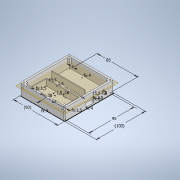
# Autodesk Inventor part: Senzor-case-new
Saved by Autodesk Inventor 2022 (Build 260153000, 153)
## iProperties
Created: 2023-05-16
Part Number: Senzor-case-new
Material: Všeobecné
Document SubType Name: Modeling
Designer: Tada
Density: 1 g/cm^3
Appearance: Výchozí
Author: Tada
Autodesk Inventor part; units mm, degrees
ref_plane "YZ Plane" through (0, 0, 0) normal (1, 0, 0) x (0, 1, 0)
ref_plane "XZ Plane" through (0, 0, 0) normal (0, 1, 0) x (-1, 0, 0)
ref_plane "XY Plane" through (0, 0, 0) normal (0, 0, 1) x (1, 0, 0)
sketch "Náčrt1" plane through (0, 0, 0) normal (0, 1, 0) x (-1, 0, 0)
  line L0 (0, 0) -> (-85, 0)
  line L1 (-85, 0) -> (-85, -95)
  line L2 (-85, -95) -> (0, -95)
  line L3 (0, -95) -> (0, 0)
  line L4 (4, 4) -> (-89, 4)
  line L5 (-89, 4) -> (-89, -99)
  line L6 (-89, -99) -> (4, -99)
  line L7 (4, -99) -> (4, 4)
  line L8 (0, 0) -> (-68, 0)
  line L9 (0, -38) -> (0, 0)
  line L10 (0, 0) -> (-69.5, 0)
  line L11 (0, -39.5) -> (0, 0)
  line L12 (0, -57.5) -> (-69.5, -57.5)
  line L13 (-85, -57.5) -> (-85, -59)
  line L14 (-69.5, -59) -> (0, -59)
  line L15 (0, -59) -> (0, -57.5)
  line L16 (-69.5, -57.5) -> (-69.5, -59)
  circle A0 centre (-77, -71.5) radius 1.25
  circle A1 centre (-77, -87) radius 1.25
  line L17 (0, 0) -> (-68, 0)
  line L18 (0, -38) -> (0, 0)
  line L19 (-7, 0) -> (-78, 0)
  line L20 (-78, 0) -> (-78, -39.5)
  line L21 (-78, -39.5) -> (-7, -39.5)
  line L22 (-7, -39.5) -> (-7, 0)
  line L23 (-8.5, 0) -> (-76.5, 0)
  line L24 (-76.5, 0) -> (-76.5, -38)
  line L25 (-76.5, -38) -> (-8.5, -38)
  line L26 (-8.5, -38) -> (-8.5, 0)
  point P0 (0, -59)
  dimension "d0" = 4
  dimension "d1" = 4
  dimension "d2" = 4
  dimension "d3" = 4
  dimension "d4" = 85
  dimension "d5" = 95
  dimension "d10" = 1.5
  dimension "d12" = 69.5
  dimension "d13" = 2.5
  dimension "d14" = 2.5
  dimension "d15" = 15.5
  dimension "d16" = 8
  dimension "d17" = 8
  dimension "d18" = 8
  dimension "d89" = 1.5
  dimension "d90" = 1.5
  dimension "d91" = 18
  dimension "d92" = 68
  dimension "d93" = 38
  dimension "d94" = 1.5
  dimension "d95" = 7
  dimension "d105" = 93
  dimension "d106" = 103
  constraints: 54 end point, 9 parallel, 7 horizontal, 6 point on line, 5 perpendicular, 2 centre point, 1 vertical
  measures "d0" distance between parallel lines of L7 L3
  measures "d1" distance between parallel lines of L6 L2
  measures "d2" distance between parallel lines of L1 L5
  measures "d3" distance between parallel lines of L4 L0
  measures "d4" distance of L1.end L2.end
  measures "d5" distance of L0.end L1.end
  measures "d10" distance between parallel lines of L12 L14
  measures "d12" distance between parallel lines of L3 L16
  measures "d13" diameter of A1
  measures "d14" diameter of A0
  measures "d15" distance of A1.centre A0.centre
  measures "d16" distance from line of L1 A1.centre
  measures "d17" distance from line of L2 A1.centre
  measures "d18" distance from line of L1 A0.centre
  measures "d89" distance between parallel lines of L25 L21
  measures "d90" distance between parallel lines of L24 L20
  measures "d91" distance between parallel lines of L12 L21
  measures "d92" distance between parallel lines of L24 L26
  measures "d93" distance between parallel lines of L10 L25
  measures "d94" distance between parallel lines of L22 L26
  measures "d95" distance between parallel lines of L3 L22
  measures "d105" distance of L4.start L4.end
  measures "d106" distance of L4.end L5.end
extrude "Vysunutí1" add sketch "Náčrt1" along normal blind 3 contours L3 L12 L16 L14 L2 L1 L0 L20 L21 L22 | L22 L21 L20 L0 L24 L25 L26 | L26 L25 L24 L0 | L3 L14 L16 L12 | A0 | A1
extrude "Vysunutí2" add sketch "Náčrt1" along normal blind 24 contours L7 L6 L5 L4
sketch "Náčrt2" plane through (0, 24, 0) normal (0, 1, 0) x (1, 0, 0)
  line L0 (-4, 99) -> (-4, -4) projected
  line L1 (-4, -4) -> (4, -4)
  line L2 (4, -4) -> (4, 4)
  line L3 (4, 4) -> (-4, 4)
  line L4 (-4, 4) -> (-4, -4)
  circle A0 centre (0, 0) radius 1.6
  line L5 (-4, -4) -> (89, -4) projected
  line L6 (42.5, -4) -> (42.5, 47.5) construction
  line L7 (4, 99) -> (-4, 99)
  line L8 (-4, 99) -> (-4, 91)
  line L9 (-4, 91) -> (4, 91)
  circle A1 centre (0, 95) radius 1.6
  line L10 (4, 91) -> (4, 99)
  line L11 (-4, 47.5) -> (42.5, 47.5) construction
  line L12 (81, 99) -> (81, 91)
  line L13 (81, 91) -> (89, 91)
  circle A2 centre (85, 95) radius 1.6
  line L14 (89, 99) -> (81, 99)
  line L15 (89, 91) -> (89, 99)
  circle A3 centre (85, 0) radius 1.6
  line L16 (81, 4) -> (81, -4)
  line L17 (81, -4) -> (89, -4)
  line L18 (89, -4) -> (89, 4)
  line L19 (89, 4) -> (81, 4)
  point P0 (0, 0)
  dimension "d28" = 8
  dimension "d29" = 8
  dimension "d30" = 3.2
  dimension "d31" = 4
  dimension "d32" = 4
  dimension "d44" = 95
  dimension "d51" = 85
  dimension "d58" = 85
  constraints: 36 end point, 4 centre point, 4 horizontal, 2 midpoint, 2 parallel, 2 vertical, 1 perpendicular, 30 other
  measures "d28" distance between parallel lines of L1 L3
  measures "d29" distance of L2.end L3.end
  measures "d30" diameter of A0
  measures "d31" distance from line of L0 A0.centre
  measures "d32" distance from line of L1 A0.centre
  measures "d44" distance of L2.end L7.start
  measures "d51" distance of L7.end L12.start
  measures "d58" distance of A0.centre A3.centre
extrude "Vysunutí5" add sketch "Náčrt2" against normal blind 12 contours L3 L2 L1 L0
extrude "Vysunutí6" add sketch "Náčrt2" against normal blind 12 contours L7 L10 L9 L0 | A0 | L16 L19 L18 L5 | L14 L15 L13 L12 | A2
ref_plane "Pracovní rovina1" through (0, 18, 0) normal (0, 1, 0) x (1, 0, 0)
sketch "Náčrt3" plane through (0, 18, 0) normal (0, 1, 0) x (1, 0, 0)
  line L0 (0, 0) -> (4, 0) projected
  line L1 (-2.825, -1.631) -> (-2.825, 1.631)
  line L2 (-2.825, 1.631) -> (0, 3.262)
  line L3 (0, 3.262) -> (2.825, 1.631)
  line L4 (2.825, 1.631) -> (2.825, -1.631)
  line L5 (-2.825, -1.631) -> (-2.825, -4)
  line L6 (-4, -4) -> (89, -4) projected
  line L7 (2.825, -1.631) -> (2.825, -4)
  line L8 (42.5, -4) -> (42.5, 45.9441) construction
  line L9 (-4, 99) -> (-4, -4) projected
  line L10 (-4, 47.5) -> (20.7945, 47.5) construction
  line L11 (-2.825, 96.631) -> (-2.825, 93.369)
  line L12 (-2.825, 93.369) -> (0, 91.738)
  line L13 (0, 91.738) -> (2.825, 93.369)
  line L14 (2.825, 93.369) -> (2.825, 96.631)
  line L15 (-2.825, 96.631) -> (-2.825, 99)
  line L16 (2.825, 96.631) -> (2.825, 99)
  line L17 (82.175, 96.631) -> (82.175, 99)
  line L18 (82.175, 96.631) -> (82.175, 93.369)
  line L19 (82.175, 93.369) -> (85, 91.738)
  line L20 (85, 91.738) -> (87.825, 93.369)
  line L21 (87.825, 93.369) -> (87.825, 96.631)
  line L22 (87.825, 96.631) -> (87.825, 99)
  line L23 (82.175, -1.631) -> (82.175, -4)
  line L24 (82.175, -1.631) -> (82.175, 1.631)
  line L25 (87.825, -1.631) -> (87.825, -4)
  line L26 (87.825, 1.631) -> (87.825, -1.631)
  line L27 (85, 3.262) -> (87.825, 1.631)
  line L28 (82.175, 1.631) -> (85, 3.262)
  line L29 (-2.825, 99) -> (2.825, 99)
  line L30 (89, 99) -> (-4, 99) projected
  line L31 (87.825, 99) -> (82.175, 99)
  line L32 (87.825, -4) -> (82.175, -4)
  point P0 (1.6, 0)
  point P1 (82.175, -4)
  point P2 (87.825, -4)
  dimension "d69" = 85
  dimension "d76" = 85
  dimension "d82" = 5.65
  constraints: 58 end point, 7 symmetric about line, 3 horizontal, 2 collinear, 2 midpoint, 2 perpendicular, 2 point on line, 2 vertical, 1 coincident, 34 other
  measures "d69" distance of L11.start L17.start
  measures "d76" distance of L1.start L23.start
  measures "d82" distance between parallel lines of L4 L1
extrude "Vysunutí7" cut sketch "Náčrt3" along normal mid plane 2.55
extrude "Vysunutí8" cut sketch "Náčrt2" against normal blind 12 contours A1 | A2 | A3
extrude "Vysunutí9" cut sketch "Náčrt2" against normal blind 12 contours A0
fillet "Zaoblení1" radius 2 4 edges at (89, 12, 4) (89, 12, -99) (-4, 12, -99) (-4, 12, 4)
extrude "Vysunutí10" add sketch "Náčrt1" along normal blind 8 contours A0 | A1
extrude "Vysunutí11" add sketch "Náčrt1" along normal blind 16 contours L22 L21 L20 L0 L24 L25 L26 | L3 L14 L16 L12
sketch "Náčrt4" plane through (85, 3, -95) normal (-1, 0, 0) x (0, 0, 1)
  line L0 (95, 0) -> (0, 0) projected
  line L1 (37.5, 0) -> (55.5, 0)
  line L2 (55.5, 0) -> (55.5, 8)
  line L3 (55.5, 8) -> (37.5, 8)
  line L4 (37.5, 8) -> (37.5, 0)
  line L5 (95, 0) -> (95, 9) projected
  point P0 (95, -3)
  dimension "d100" = 39.5
  dimension "d101" = 18
  dimension "d102" = 8
  constraints: 8 end point, 2 parallel, 1 horizontal, 1 perpendicular, 1 point on line
  measures "d100" distance between parallel lines of L5 L2
  measures "d101" distance between parallel lines of L4 L2
  measures "d102" distance between parallel lines of L3 L0
extrude "Vysunutí12" cut sketch "Náčrt4" against normal blind 16
equation "\"d1\" = d0"
equation "\"d2\" = d0"
equation "\"d3\" = d0"
equation "\"d14\" = d13"
equation "\"d18\" = d16"
equation "\"d90\" = d89"
equation "\"d94\" = d89"
equation "\"d29\" = d28"
equation "\"d32\" = d31"
